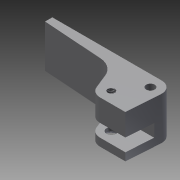
# Autodesk Inventor part: D-037
Saved by Autodesk Inventor 2015 (Build 190159000, 159)
## iProperties
Company: MARCHA TECHNOLOGY
Created: 2013-10-24
Part Number: D-037
Document SubType Name: Modeling
Designer: O.Martin
Density: 1 g/cm^3
Project: WITBOXprinter_K01
Description: PALANCA EXTRUDER
Stock Number: 28655
Mass: 2.84259 g
Surface Area: 22.7646 cm^2
Volume: 2.84259 cm^3
Material: Generic
Appearance: Light Gray
Author: O.Martin
Autodesk Inventor part; units mm, degrees
ref_plane "YZ Plane" through (0, 0, 0) normal (1, 0, 0) x (0, 1, 0)
ref_plane "XZ Plane" through (0, 0, 0) normal (0, 1, 0) x (-1, 0, 0)
ref_plane "XY Plane" through (0, 0, 0) normal (0, 0, 1) x (1, 0, 0)
sketch "Boceto1" plane through (0, 0, 0) normal (0, 0, 1) x (1, 0, 0)
  circle A0 centre (0, 0) radius 6.25 construction
  circle A1 centre (17.25, 8) radius 1.5
  arc A2 (21.25, 8) -> (17.25, 12) centre (17.25, 8) ccw
  circle A3 centre (11.5, 0) radius 5 construction
  line L0 (0, 0) -> (0, -26.8639) construction
  arc A4 (17.25, 12) -> (17.25, 12) centre (17.25, 8) ccw
  line L1 (17.25, 12) -> (-21.25, 12)
  line L2 (-21.25, 12) -> (-21.25, 9.4506)
  line L3 (11.5, -4) -> (21.25, -4)
  line L4 (21.25, -4) -> (21.25, 8)
  circle A5 centre (11.5, 0) radius 1
  line L5 (-0.2617, 7.9829) -> (-21.25, 9.4506)
  arc A6 (5.7482, 3.6026) -> (-0.2617, 7.9829) centre (-0.75, 1) ccw
  line L6 (5.7482, 3.6026) -> (7.7868, -1.4872)
  arc A7 (7.7868, -1.4872) -> (11.5, -4) centre (11.5, 0) ccw
  dimension "d0" = 3
  dimension "d5" = 17.25
  dimension "d9" = 10
  dimension "d78" = 42.5
  dimension "d79" = 2
  dimension "d112" = 12.5
  dimension "d113" = 8
  dimension "d115" = 16
  dimension "d116" = 4
  dimension "d117" = 4
  dimension "d118" = 7
  dimension "d120" = 0
  dimension "d121" = 11.5
  dimension "d122" = 0.75
  dimension "d123" = 1
  constraints: 14 end point, 8 centre point, 8 point on circle, 7 tangent, 4 coincident, 4 perpendicular, 1 concentric, 1 horizontal
  measures "d0" diameter of A1
  measures "d5" horizontal distance of A1.centre A0.centre
  measures "d9" diameter of A3
  measures "d78" distance between parallel lines of L4 L2
  measures "d79" diameter of A5
  measures "d112" diameter of A0
  measures "d113" vertical distance of A1.centre A0.centre
  measures "d115" distance between parallel lines of L3 L1
  measures "d116" distance from line of L1 A1.centre
  measures "d117" angle of L1 L5
  measures "d118" radius of A6
  measures "d120" vertical distance of A3.centre A0.centre
  measures "d121" distance of A0.centre A3.centre
  measures "d122" horizontal distance of A6.centre A0.centre
  measures "d123" vertical distance of A0.centre A6.centre
extrude "Extrusión1" add sketch "Boceto1" along normal mid plane 15
sketch "Boceto6" plane through (21.25, -4, 7.5) normal (1, 0, 0) x (0, 0, -1)
  line L0 (0, 0) -> (15, 0) projected
  line L1 (15, 0) -> (15, 12) projected
  line L2 (12.25, 0) -> (7.75, 0)
  line L3 (7.75, 0) -> (7.75, 9.5)
  line L4 (7.75, 9.5) -> (12.25, 9.5)
  line L5 (12.25, 9.5) -> (12.25, 0)
  line L6 (0, 3) -> (0, 5) projected
  line L7 (0, 4) -> (4.0286, 4) construction
  line L8 (0, 12) -> (15, 12) projected
  line L9 (10, 9.5) -> (10, 1.1664) construction
  point P0 (15, 9.5)
  dimension "d81" = 5.5
  dimension "d83" = 4.5
  dimension "d129" = 5
  constraints: 12 end point, 3 perpendicular, 2 midpoint, 2 parallel, 1 horizontal, 1 point on line
  measures "d81" distance between parallel lines of L4 L7
  measures "d83" distance between parallel lines of L3 L5
  measures "d129" distance between parallel lines of L1 L9
extrude "Extrusión7" cut sketch "Boceto6" against normal through all
hole "Agujero5" at (11.5, 0, -7.5) direction (0, 0, 1) diameter 3.4 depth 5 tip angle 118 countersink diameter 6.3 countersink angle 90 clearance for "Tornillo de cabeza avellanada con resalte ISO 2010" size "M3" standard "DIN"
hole "Agujero6" at (11.5, 0, 7.5) direction (0, 0, -1) diameter 2.459 depth 10 tip angle 118 thread size "M3x0.5" class "6H" standard "ISO Metric profile"
sketch "Boceto7" plane through (-21.25, 12, 7.5) normal (0, 1, 0) x (1, 0, 0)
  line L0 (38.5, 15) -> (38.5, 0) projected
  line L1 (38.5, 15) -> (0, 15) projected
  circle A0 centre (27.25, 10) radius 1.5
  dimension "d105" = 5
  dimension "d106" = 3
  dimension "d107" = 11.25
  constraints: 1 centre point
  measures "d105" distance from line of L1 A0.centre
  measures "d106" diameter of A0
  measures "d107" distance from line of L0 A0.centre
extrude "Extrusión8" cut sketch "Boceto7" against normal through all
sketch "Boceto8" plane through (0, 0, 7.5) normal (0, 0, 1) x (1, 0, 0)
  line L0 (21.25, 8) -> (21.25, -4) projected
  arc A0 (21.25, 8) -> (17.25, 12) centre (17.25, 8) ccw projected
  line L1 (-0.2617, 7.9829) -> (-21.25, 9.4506) projected
  line L2 (21.25, -4) -> (11.5, -4) projected
  circle A1 centre (17.25, 8) radius 4
  line L3 (21.2403, 7.721) -> (20.4206, -4)
  constraints: 2 end point, 2 point on circle, 1 centre point, 1 coincident, 1 perpendicular, 1 point on line, 1 tangent
extrude "Extrusión9" cut sketch "Boceto8" against normal through all contours L0 L2 L3 A1
chamfer "Chaflán4" distance 1.5 angle 45 1 edges at (4.5, 12, -2.5)
sketch "Boceto2" plane through (0, 0, 7.5) normal (0, 0, 1) x (1, 0, 0)
  circle A0 centre (11.875, 0) radius 4 projected
  point P0 (7.875, 0)
  point P1 (11.875, -4)
  constraints: 1 coincident
sketch "Boceto3" plane through (0, 0, -7.5) normal (0, 0, -1) x (-1, 0, 0)
  circle A0 centre (-11.875, 0) radius 4 projected
  point P0 (-11.5, -4)
  point P1 (-7.875, 0)
  constraints: 1 coincident, 1 other
sketch "Boceto4" plane through (16.971, 11.9903, 7.5) normal (-0.0697565, 0.9975641, 0) x (0.9975641, 0.0697565, 0)
  line L0 (0, 0) -> (0, 15)
  circle A0 centre (-11.2807, 7.5) radius 2
  line L1 (-39, 0) -> (0, 0) projected
  line L2 (0, 15) -> (0, 0) projected
  line L3 (0, 15) -> (-39, 15) projected
  line L4 (-39, 15) -> (-39, 0) projected
  point P0 (0, 7.5)
  dimension "d52" = 4
  constraints: 2 end point, 1 centre point, 1 horizontal alignment, 1 midpoint
  measures "d52" diameter of A0
sketch "Boceto5" plane through (16.971, 11.9903, 7.5) normal (-0.0697565, 0.9975641, 0) x (0.9975641, 0.0697565, 0)
  line L0 (0, 15) -> (0, 0) projected
  line L1 (4, 15) -> (4, 0) projected
  point P0 (-11.25, 7.5)
  point P1 (0, 7.5)
  dimension "d67" = 15.25
  constraints: 1 horizontal alignment, 1 midpoint
  measures "d67" distance from line of L1 point (-11.25, 7.5)
body "Solid1"
